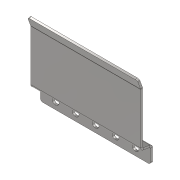
# Autodesk Inventor part: SlipersLåda 211018011
Saved by Autodesk Inventor 2020 (Build 240168000, 168)
## iProperties
Created: 2021-10-20
Part Number: SlipersLåda 211018011
Material: Steel, Mild
Document SubType Name: Sheet Metal
Designer: dicpet001
Density: 7.85 g/cm^3
Sheet Metal Rule: Default_mm
Appearance: Semi-Polished
Flat Pattern Width: 8.68012 cm
Flat Pattern Length: 11 cm
Flat Pattern Area: 95.4813 cm^2
Sheet Metal Width: 86,801 mm
Sheet Metal Length: 110,000 mm
Sheet Metal Area: 9548,127 mm^2
Author: dicpet001
Autodesk Inventor part; units mm, degrees
ref_plane "YZ Plane" through (0, 0, 0) normal (1, 0, 0) x (0, 1, 0)
ref_plane "XZ Plane" through (0, 0, 0) normal (0, 1, 0) x (-1, 0, 0)
ref_plane "XY Plane" through (0, 0, 0) normal (0, 0, 1) x (1, 0, 0)
sketch "Sketch1" plane through (0, 0, 0) normal (0, 0, 1) x (1, 0, 0)
  line L0 (0, 10.5) -> (0, -10.5)
  line L1 (-77, 0) -> (77, 0)
  line L2 (-55, 7.5) -> (55, 7.5)
  line L3 (55, 7.5) -> (55, -7.5)
  line L4 (55, -7.5) -> (-55, -7.5)
  line L5 (-55, -7.5) -> (-55, 7.5)
  point P0 (0, 0)
  dimension "d0" = 110
  dimension "d1" = 15
  measures "d0" distance of L3.end L4.end
  measures "d1" distance of L4.end L2.start
extrude "Plate1" add sketch "Sketch1" against normal blind 2
sketch "Sketch2" plane through (-55, 7.5, 0) normal (0, 0.9848078, -0.1736482) x (-1, 0, 0)
  line L0 (-110, 0) -> (0, 0)
  line L1 (0, 0) -> (0, 8.3218)
  line L2 (0, 8.3218) -> (-110, 8.3218)
  line L3 (-110, 8.3218) -> (-110, 0)
  constraints: 6 end point, 1 horizontal, 1 perpendicular, 1 vertical
edge flange "Flange1" height 10 angle 80 thickness 2 bend radius 1 thickness toward (0, 0.9848078, -0.1736482) relief tear relief width 2 relief depth 1 edges at (0, 7.5, 0) wall of the first edge with corners at (55, 7.5, 0) (-55, 7.5, 0) (-55, 8.9451, 8.1954) (55, 8.9451, 8.1954)
bend "Bend1"
corner "Corner1"
sketch "Sketch3" plane through (55, 10.9147, 7.8481) normal (0, 0, 1) x (1, 0, 0)
  line L0 (-110, 0) -> (0, 0)
  line L1 (0, 0) -> (0, 61.5858)
  line L2 (0, 61.5858) -> (-110, 61.5858)
  line L3 (-110, 61.5858) -> (-110, 0)
  constraints: 6 end point, 1 horizontal, 1 perpendicular, 1 vertical
edge flange "Flange2" height 63.264 angle 80 thickness 2 bend radius 1 thickness toward (0, 0, 1) relief tear relief width 2 relief depth 1 edges at (0, 10.9147, 7.8481) wall of the first edge with corners at (-55, 10.9147, 7.8481) (55, 10.9147, 7.8481) (55, 72.5005, 7.8481) (-55, 72.5005, 7.8481)
bend "Bend2"
corner "Corner2"
sketch "Sketch4" plane through (0, 0, 0) normal (0, 0, 1) x (1, 0, 0)
  line L0 (55, 6.6609) -> (-55, 6.6609) projected
  line L1 (-55, -7.5) -> (-55, 6.6609) projected
  line L2 (55, -7.5) -> (-55, -7.5) projected
  line L3 (55, 6.6609) -> (55, -7.5) projected
  circle A0 centre (0, 0) radius 3.5
  circle A1 centre (-20, 0) radius 3.5
  circle A2 centre (-40, 0) radius 3.5
  circle A3 centre (20, 0) radius 3.5
  circle A4 centre (40, 0) radius 3.5
  dimension "d23" = 7
  dimension "d26" = 20
  dimension "d33" = 20
  constraints: 5 centre point, 2 horizontal, 1 coincident, 8 other
  measures "d23" diameter of A0
  measures "d26" distance of A0.centre A1.centre
  measures "d33" distance of A0.centre A3.centre
extrude "Cut1" cut sketch "Sketch4" against normal blind 2 contours A0 | A1 | A2 | A3 | A4
fillet "Fillet1" radius 2 4 edges at (-55, 72.5005, 8.8481) (55, 72.5005, 8.8481) (-55, -7.5, -1) (55, -7.5, -1)
sketch "Sketch5" plane through (-55, 11.7538, 9.8481) normal (0, 0, 1) x (1, 0, 0)
  arc A0 (110, 58.7467) -> (108, 60.7467) centre (108, 58.7467) ccw projected
  line L0 (2, 60.7467) -> (108, 60.7467) projected
  arc A1 (2, 60.7467) -> (0, 58.7467) centre (2, 58.7467) ccw projected
  line L1 (0, 0) -> (0, 58.7467) projected
  line L2 (0, 0) -> (110, 0) projected
  line L3 (110, 58.7467) -> (110, 0) projected
  line L4 (0, 0) -> (0, 58.7467) projected
  line L5 (0, 50.7467) -> (110, 50.7467)
  point P0 (55, -11.7538)
  dimension "d41" = 10
  constraints: 2 end point, 2 point on line, 1 perpendicular
  measures "d41" distance between parallel lines of L0 L5
fold "Fold1" angle 20 bend radius 1 thickness 2 k factor 0.44 line from (-55, 62.5005, 9.8481) to (55, 62.5005, 9.8481) line at bend start moving side (0, 1, 0) folds toward (0, 0, 1)
equation "\"d38\" = Thickness"
equation "\"d2\" = Thickness"
equation "\"d42\" = BendReliefWidth"
equation "\"d43\" = BendReliefDepth"
equation "\"d44\" = MinimumRemnant"
equation "\"d45\" = TransitionRadius"
equation "\"d3\" = BendReliefWidth"
equation "\"d4\" = BendReliefDepth"
equation "\"d5\" = MinimumRemnant"
equation "\"d6\" = TransitionRadius"
equation "\"d10\" = CornerReliefSize"
equation "\"d11\" = GapSize"
equation "\"d12\" = JacobiRadiusSize"
equation "\"d13\" = BendReliefWidth"
equation "\"d14\" = BendReliefDepth"
equation "\"d15\" = MinimumRemnant"
equation "\"d16\" = TransitionRadius"
equation "\"d20\" = CornerReliefSize"
equation "\"d21\" = GapSize"
equation "\"d22\" = JacobiRadiusSize"
equation "\"BendRadius\" = Thickness"
equation "\"BendReliefWidth\" = Thickness"
equation "\"BendReliefDepth\" = 0.5 * Thickness"
equation "\"CornerReliefSize\" = 4 * Thickness"
equation "\"MinimumRemnant\" = 2 * Thickness"
equation "\"TransitionRadius\" = BendRadius"
equation "\"JacobiRadiusSize\" = BendRadius"
equation "\"GapSize\" = Thickness"
equation "\"Thickness\" = 2"
body "Solid1"
